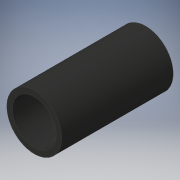
# Autodesk Inventor part: DPLX_P034_RPS VIPE Viton Insualtion
Saved by Autodesk Inventor 2018 (Build 220112000, 112)
## iProperties
Created: 2018-04-27
Part Number: DPLX_P034_RPS VIPE Viton Insualtion
Material: Rubber, Silicone
Document SubType Name: Modeling
Designer: R.P.SMITH
Mass: 22.307 g
Surface Area: 118.034 cm^2
Volume: 17.8456 cm^3
Density: 1.25 g/cm^3
Appearance: Rubber - Black
Author: R.P.SMITH
Autodesk Inventor part; units mm, degrees
ref_plane "YZ Plane" through (0, 0, 0) normal (1, 0, 0) x (0, 1, 0)
ref_plane "XZ Plane" through (0, 0, 0) normal (0, 1, 0) x (-1, 0, 0)
ref_plane "XY Plane" through (0, 0, 0) normal (0, 0, 1) x (1, 0, 0)
sketch "Sketch1" plane through (0, 0, 0) normal (0, 0, 1) x (1, 0, 0)
  circle A0 centre (0, 0) radius 12.5
  circle A1 centre (0, 0) radius 15.675
  dimension "d0" = 25
  dimension "d1" = 3.175
  constraints: 2 centre point, 1 coincident
  measures "d0" diameter of A0
  measures "d1" radial gap between concentric circles of A0 A1
extrude "Extrusion1" add sketch "Sketch1" along normal mid plane 63.5
body "Solid1"
